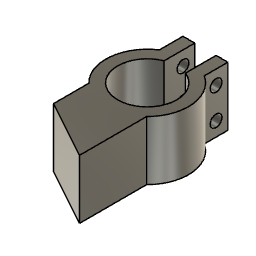
motor clamp assembly v6 (Autodesk Fusion 360 archive; units mm, degrees)
design "clamp"
Autodesk Fusion 360 part; units mm, degrees
sketch "Sketch1" plane through (0, 0, 0) normal (0, 0, 1) x (1, 0, 0)
  circle A0 centre (0, 0) radius 12.5
  circle A1 centre (0, 0) radius 17.5
  line L0 (-9.525, 14.6807) -> (9.525, 14.6807)
  line L1 (-4.525, 11.6522) -> (-9.525, 11.6522)
  line L2 (-9.525, 11.6522) -> (-9.525, 24.6807)
  line L3 (-9.525, 24.6807) -> (-4.525, 24.6807)
  line L4 (-4.525, 24.6807) -> (-4.525, 11.6522)
  line L5 (4.525, 11.6522) -> (9.525, 11.6522)
  line L6 (9.525, 11.6522) -> (9.525, 24.6807)
  line L7 (9.525, 24.6807) -> (4.525, 24.6807)
  line L8 (4.525, 24.6807) -> (4.525, 11.6522)
  line L9 (0.0006, -27.5) -> (12.2475, -27.5)
  line L10 (12.2475, -27.5) -> (12.2475, -12.5)
  line L11 (12.2475, -12.5) -> (0.0006, -12.5)
  line L12 (0.0006, -12.5) -> (0.0006, -27.5)
  line L13 (-12.2462, -27.5) -> (-12.2462, -12.5)
  line L14 (0.0006, -27.5) -> (-12.2462, -27.5)
  line L15 (-12.2462, -12.5) -> (0.0006, -12.5)
  line L16 (12.2475, -27.5) -> (12.2475, -41)
  line L17 (12.2475, -41) -> (-12.2462, -27.5)
  dimension "d1" = 25
  dimension "d2" = 35
  dimension "d3" = 19.05
  dimension "d4" = 10
  dimension "d5" = 5
  dimension "d6" = 5
  dimension "d7" = 10
  dimension "d18" = 12.2468
  dimension "d19" = 15
  dimension "d27" = 13.5
  constraint coincident A0.centre A1.centre
  constraint coincident A1 L0.start
  constraint coincident A1 L0.end
  constraint horizontal L0
  constraint horizontal L1
  constraint vertical L2
  constraint horizontal L3
  constraint vertical L4
  constraint coincident A0 L1.start
  constraint horizontal L5
  constraint vertical L6
  constraint horizontal L7
  constraint vertical L8
  constraint coincident A0 L5.start
  constraint coincident L0.end L6
  constraint coincident L0.start L2
  constraint horizontal L9
  constraint vertical L10
  constraint horizontal L11
  constraint vertical L12
  constraint coincident A1 L10.end
  constraint coincident A0 L11.end
  constraint symmetric L9.start L12 L14.start
  constraint symmetric L9.end L12 L13.start
  constraint symmetric L10.end L12 L13.end
  constraint symmetric L11.end L12 L15.end
  constraint perpendicular L9 L16
  measures "d1" diameter of A0
  measures "d2" diameter of A1
  measures "d3" distance of L0.start L0.end
  measures "d4" distance of L0.start L2.end
  measures "d5" distance of L2.end L3.end
  measures "d6" distance of L5.start L5.end
  measures "d7" distance of L0.end L6.end
  measures "d18" distance of L9.start L9.end
  measures "d19" distance of L9.end L10.end
  measures "d27" distance of L9.end L16.end
extrude "Extrude1" add sketch "Sketch1" along normal blind 25 contours A0 A1 L5 L6 L11 | L0 L5 L6 L8 | A0 A1 L1 L2 L15 | A1 L11 L12 | A1 L12 L15 | L0 L1 L2 L4 | A1 L0 L8 | A1 L9 L10 L12 | A1 L12 L13 L14 | A1 L0 L4 | A1 L6 L7 L8 | L9 L14 L16 L17 | A1 L2 L3 L4
hole "Hole1" at (9.525, 19.6807, 19) direction (-1, 0, 0) diameter 5 depth 20 tip angle 180
hole "Hole2" at (-9.525, 19.6807, 6) direction (1, 0, 0) diameter 5 depth 20 tip angle 180
equation "d6 = d5"
equation "d7 = d4"
